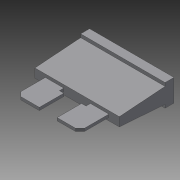
# Autodesk Inventor part: ATCFuse
Saved by Autodesk Inventor 2014 SP1 (Build 180222100, 222)
## iProperties
Created: 2016-03-18
Part Number: ATCFuse
Material: Generic
Document SubType Name: Modeling
Designer: Tyler
Density: 1 g/cm^3
Appearance: Default
Author: Tyler
Autodesk Inventor part; units mm, degrees
ref_plane "YZ Plane" through (0, 0, 0) normal (1, 0, 0) x (0, 1, 0)
ref_plane "XZ Plane" through (0, 0, 0) normal (0, 1, 0) x (-1, 0, 0)
ref_plane "XY Plane" through (0, 0, 0) normal (0, 0, 1) x (1, 0, 0)
sketch "Sketch1" plane through (0, 0, 0) normal (0, 0, 1) x (1, 0, 0)
  line L0 (-9.5, 12.3) -> (9.5, 12.3)
  line L1 (9.5, 12.3) -> (9.5, 0)
  line L2 (9.5, 0) -> (-9.5, 0)
  line L3 (-9.5, 0) -> (-9.5, 12.3)
  line L4 (-9.5, 12.3) -> (9.5, 0) construction
  line L5 (9.5, 12.3) -> (-9.5, 0) construction
  point P0 (0, 0)
  point P1 (0, 6.15)
  dimension "d0" = 12.3
  dimension "d1" = 19
  dimension "d2" = 0
  dimension "d3" = 12.3
  constraints: 12 end point, 2 midpoint, 2 parallel, 1 horizontal, 1 perpendicular
  measures "d0" distance of L2.end L0.start
  measures "d1" distance of L0.start L0.end
  measures "d2" horizontal distance of point (0, 0) point (0, 6.15)
  measures "d3" distance from line of point (0, 0) L0
extrude "Extrusion1" add sketch "Sketch1" along normal mid plane 5
sketch "Sketch2" plane through (0, 0, 0) normal (0, 0, 1) x (1, 0, 0)
  line L0 (-7.15, 1) -> (-7.15, -5.5)
  line L1 (-6.15, -6.5) -> (-2, -6.5)
  line L2 (-2, -6.5) -> (-2, -1)
  line L3 (-2, -1) -> (-3, -1)
  line L4 (-3, -1) -> (-3, 1)
  line L5 (-3, 1) -> (-7.15, 1)
  line L6 (-9.5, 0) -> (9.5, 0) projected
  line L7 (0, 0) -> (0, 7.1725) construction
  line L8 (-7.15, -5.5) -> (-6.15, -6.5)
  line L9 (7.15, 1) -> (7.15, -5.5)
  line L10 (6.15, -6.5) -> (2, -6.5)
  line L11 (2, -6.5) -> (2, -1)
  line L12 (2, -1) -> (3, -1)
  line L13 (3, -1) -> (3, 1)
  line L14 (3, 1) -> (7.15, 1)
  line L15 (7.15, -5.5) -> (6.15, -6.5)
  point P0 (-7.15, -6.5)
  point P1 (7.15, -6.5)
  dimension "d6" = 6.5
  dimension "d7" = 2
  dimension "d8" = 7.15
  dimension "d9" = 1
  dimension "d10" = 1
  dimension "d11" = 1
  dimension "d12" = 1
  dimension "d13" = 1
  constraints: 30 end point, 8 symmetric about line, 4 parallel, 4 point on line, 2 perpendicular, 1 vertical
  measures "d6" distance between parallel lines of L1 L6
  measures "d7" distance between parallel lines of L7 L2
  measures "d8" distance between parallel lines of L7 L0
  measures "d9" distance of L2.end L3.end
  measures "d10" distance between parallel lines of L6 L3
  measures "d11" distance of L0.end point (-7.15, -6.5)
  measures "d12" distance of L1.start point (-7.15, -6.5)
  measures "d13" distance between parallel lines of L6 L5
extrude "Extrusion2" add sketch "Sketch2" along normal mid plane 0.64
sketch "Sketch3" plane through (9.5, 0, 2.5) normal (1, 0, 0) x (0, 0, -1)
  line L0 (0, 12.3) -> (5, 12.3) projected
  line L1 (0, 0) -> (0, 12.3) projected
  line L2 (0, 0) -> (5, 0) projected
  line L3 (5, 12.3) -> (5, 0) projected
  line L4 (-1.5, 10.3) -> (0.75, 10.3)
  line L5 (0.75, 10.3) -> (1.5, 0)
  line L6 (-1.5, 10.3) -> (-1.5, -2)
  line L7 (-1.5, -2) -> (1.5, -2)
  line L8 (1.5, -2) -> (1.5, 0)
  line L9 (2.5, 0) -> (2.5, 10.8693) construction
  line L10 (6.5, 10.3) -> (4.25, 10.3)
  line L11 (4.25, 10.3) -> (3.5, 0)
  line L12 (6.5, 10.3) -> (6.5, -2)
  line L13 (6.5, -2) -> (3.5, -2)
  line L14 (3.5, 0) -> (3.5, -2)
  dimension "d16" = 2
  dimension "d17" = 0.75
  dimension "d18" = 1.5
  dimension "d19" = 2
  dimension "d20" = 1.5
  constraints: 22 end point, 5 symmetric about line, 4 perpendicular, 2 parallel, 1 point on line
  measures "d16" distance between parallel lines of L4 L0
  measures "d17" distance from line of L1 L4.end
  measures "d18" distance between parallel lines of L1 L8
  measures "d19" distance between parallel lines of L7 L2
  measures "d20" distance between parallel lines of L6 L1
extrude "Extrusion3" cut sketch "Sketch3" against normal through all contours L4 L5 L2 L1 | L1 L2 L8 L7 L6 L4 | L10 L12 L13 L14 L2 L3 | L3 L2 L11 L10
equation "\"d3\" = d0"
equation "\"d12\" = d11"
body "Solid1"
